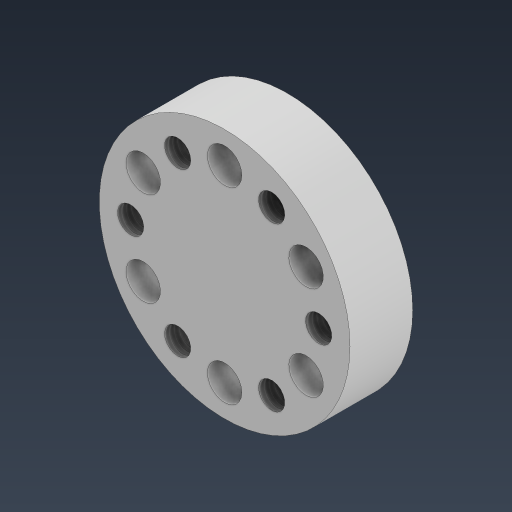
# Autodesk Inventor part: 3D Model
Saved by Autodesk Inventor 2024 (Build 280153000, 153)
## iProperties
Created: 2024-03-13
Part Number: 3D Model
Material: Genérico
Document SubType Name: Modeling
Designer: Administrator
Density: 1 g/cm^3
Appearance: Padrão
Author: Administrator
Autodesk Inventor part; units mm, degrees
ref_plane "YZ Plane" through (0, 0, 0) normal (1, 0, 0) x (0, 1, 0)
ref_plane "XZ Plane" through (0, 0, 0) normal (0, 1, 0) x (-1, 0, 0)
ref_plane "XY Plane" through (0, 0, 0) normal (0, 0, 1) x (1, 0, 0)
sketch "Esboço1" plane through (0, 0, 0) normal (0, 0, 1) x (1, 0, 0)
  circle A0 centre (0, 0) radius 40
  dimension "d0" = 80
  constraints: 1 centre point, 1 coincident
  measures "d0" diameter of A0
extrude "Extrusão1" add sketch "Esboço1" along normal blind 20
sketch "Esboço2" plane through (0, 0, 20) normal (0, 0, 1) x (1, 0, 0)
  point P0 (0, 0)
  point P1 (0, 30)
  dimension "d3" = 30
  constraints: 1 vertical alignment
  measures "d3" distance of point (0, 0) point (0, 30)
hole "Furo1" at (0, 30, 20) direction (0, 0, -1) diameter 11 end through all
pattern_circular "Padrão circular1" count 6 over 360 about axis through (0, 0, 0) along (0, 0, 1) of "Furo1"
sketch "Esboço3" plane through (0, 0, 20) normal (0, 0, 1) x (1, 0, 0)
  circle A0 centre (0, 30) radius 5.5 projected
  circle A1 centre (0, 0) radius 30 construction
  line L0 (0, 0) -> (-62.0397, 0) construction
  line L1 (0, 0) -> (-27.415, 47.4843)
  point P0 (-15, 25.9808)
  dimension "d14" = 60
  constraints: 4 end point, 2 point on circle, 1 centre point, 1 coincident, 1 horizontal, 1 point on line
  measures "d14" angle of L0 L1
hole "Furo2" at (-15, 25.9808, 20) direction (0, 0, -1) diameter 8.376 end through all thread size "M10x1.5" class "6H" standard "ISO Metric profile"
pattern_circular "Padrão circular2" count 6 over 360 about axis through (0, 0, 0) along (0, 0, 1) of "Furo2"
